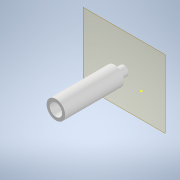
# Autodesk Inventor part: motor_casing
Saved by Autodesk Inventor 2020 (Build 240168000, 168)
## iProperties
Created: 2020-07-03
Part Number: motor_casing
Material: Generic
Document SubType Name: Modeling
Designer: Ashiqrahman
Density: 1 g/cm^3
Appearance: Default
Author: Ashiqrahman
Autodesk Inventor part; units mm, degrees
ref_plane "YZ Plane" through (0, 0, 0) normal (1, 0, 0) x (0, 1, 0)
ref_plane "XZ Plane" through (0, 0, 0) normal (0, 1, 0) x (-1, 0, 0)
ref_plane "XY Plane" through (0, 0, 0) normal (0, 0, 1) x (1, 0, 0)
ref_plane "Work Plane1" through (0, 0, 0) normal (0, 0, 1) x (1, 0, 0)
sketch "Sketch1" plane through (0, 0, 0) normal (0, 0, 1) x (1, 0, 0)
  line L0 (-17.0566, -40) -> (-17.0566, -50) projected
  line L1 (-17.0566, -50) -> (17.0566, -50) projected
  line L2 (17.0566, -50) -> (17.0566, 50) projected
  line L3 (17.0566, 50) -> (-17.0566, 50) projected
  line L4 (-17.0566, 50) -> (-17.0566, 40) projected
  line L5 (-68.8301, 40) -> (-17.0566, 40) projected
  line L6 (-68.8301, 40) -> (-68.8301, 50) projected
  line L7 (-68.8301, 50) -> (-102.9434, 50) projected
  line L8 (-102.9434, 50) -> (-102.9434, -50) projected
  line L9 (-102.9434, -50) -> (-68.8301, -50) projected
  line L10 (-68.8301, -50) -> (-68.8301, -40) projected
  line L11 (-68.8301, -40) -> (-17.0566, -40) projected
  circle A0 centre (-42.9434, 0) radius 5
  circle A1 centre (-42.9434, 0) radius 7.5
  line L12 (-46.8059, 3.175) -> (-39.0808, 3.175) construction
  line L13 (-39.0808, 3.175) -> (-39.0808, -3.175) construction
  line L14 (-39.0808, -3.175) -> (-46.8059, -3.175)
  line L15 (-46.8059, -3.175) -> (-46.8059, 3.175) construction
  line L16 (-46.8059, 3.175) -> (-39.0808, -3.175) construction
  line L17 (-39.0808, 3.175) -> (-46.8059, -3.175) construction
  point P0 (0, 0)
  dimension "d0" = 10
  dimension "d1" = 15
  constraints: 12 end point, 2 midpoint, 2 parallel, 1 centre point, 1 coincident, 1 horizontal, 1 perpendicular, 3 other
  measures "d1" diameter of A1
ref_plane "Work Plane2" through (-42.9434, 0, 15) normal (0, 0, 1) x (1, 0, 0)
sketch "Sketch2" plane through (-42.9434, 0, 15) normal (0, 0, 1) x (1, 0, 0)
  circle A0 centre (0, 0) radius 10
  circle A1 centre (0, 0) radius 7.5 projected
  point P0 (42.9434, 0)
  dimension "d4" = 20
  constraints: 1 centre point
  measures "d4" diameter of A0
extrude "Extrusion2" add sketch "Sketch2" along normal blind 10
sketch "Sketch3" plane through (-42.9434, 0, 15) normal (0, 0, -1) x (-1, 0, 0)
  point P0 (-42.9434, 0)
sketch "Sketch4" plane through (-42.9434, 0, 15) normal (0, 0, -1) x (-1, 0, 0)
  circle A0 centre (0, 0) radius 10
  circle A1 centre (0, 0) radius 15
  point P0 (-42.9434, 0)
  dimension "d7" = 30
  constraints: 2 centre point, 1 coincident
  measures "d7" diameter of A1
extrude "Extrusion3" add sketch "Sketch4" against normal blind 95
body "Solid1"
